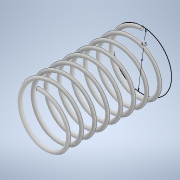
# Autodesk Inventor part: spring2
Saved by Autodesk Inventor 2022 (Build 260153000, 153)
## iProperties
Created: 2024-01-11
Part Number: spring2
Material: Generisch
Document SubType Name: Modeling
Designer: Marc Panse
Density: 1 g/cm^3
Appearance: Vorgabe
Author: Marc Panse
Autodesk Inventor part; units mm, degrees
ref_plane "YZ Plane" through (0, 0, 0) normal (1, 0, 0) x (0, 1, 0)
ref_plane "XZ Plane" through (0, 0, 0) normal (0, 1, 0) x (-1, 0, 0)
ref_plane "XY Plane" through (0, 0, 0) normal (0, 0, 1) x (1, 0, 0)
sketch "Skizze1" plane through (0, 0, 0) normal (0, 0, 1) x (1, 0, 0)
  circle A0 centre (0, 0) radius 2.25
  dimension "d0" = 4.5
  constraints: 1 centre point, 1 coincident
  measures "d0" diameter of A0
sketch "Skizze4" plane through (0, 0, 0) normal (1, 0, 0) x (0, 1, 0)
  line L0 (2.25, 0) -> (-2.25, 0) projected
  circle A0 centre (2.1101, 0) radius 0.1399
  point P0 (0, 0)
  constraints: 1 horizontal alignment, 1 point on line, 2 other
coil "Spirale1" sketch "Skizze4" operation add axis through (0, 0, -10) along (0, 0, 1) pitch 1 turns 8 hand right
